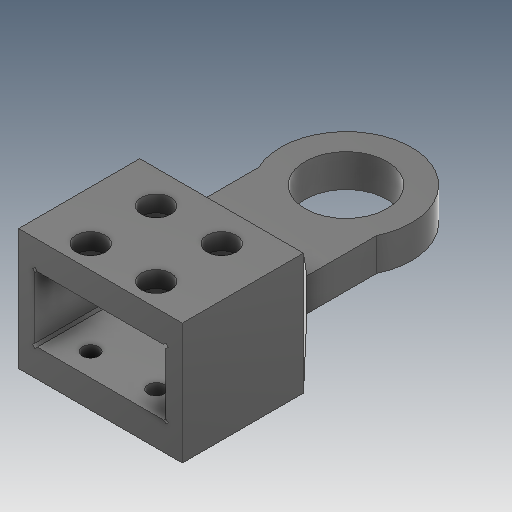
# Autodesk Inventor part: EndEffectorJoint
Saved by Autodesk Inventor 2020.3 (Build 243373000, 373)
## iProperties
Created: 2021-08-11
Part Number: EndEffectorJoint
Material: ABS Plastic
Document SubType Name: Modeling
Designer: justi
Density: 1.06 g/cm^3
Appearance: Smooth - Black
Mass: 59.7903 g
Surface Area: 233.875 cm^2
Volume: 56.4059 cm^3
Author: justi
Autodesk Inventor part; units mm, degrees
note: some values were not read from the file. Chosen so that the rebuilt part matches the saved one: direction of "Hole1".
ref_plane "YZ Plane" through (0, 0, 0) normal (1, 0, 0) x (0, 1, 0)
ref_plane "XZ Plane" through (0, 0, 0) normal (0, 1, 0) x (-1, 0, 0)
ref_plane "XY Plane" through (0, 0, 0) normal (0, 0, 1) x (1, 0, 0)
sketch "Sketch1" plane through (0, 0, 0) normal (0, 1, 0) x (-1, 0, 0)
  line L0 (25, 18.5) -> (-25, 18.5)
  line L1 (-25, 18.5) -> (-25, -18.5)
  line L2 (-25, -18.5) -> (25, -18.5)
  line L3 (25, -18.5) -> (25, 18.5)
  line L4 (25, 18.5) -> (-25, -18.5) construction
  line L5 (-25, 18.5) -> (25, -18.5) construction
  point P0 (0, 0)
  dimension "d0" = 50
  dimension "d1" = 37
  constraints: 12 end point, 2 midpoint, 2 parallel, 1 horizontal, 1 perpendicular
  measures "d0" distance of L2.end L1.end
  measures "d1" distance of L1.end L0.end
extrude "Extrusion1" add sketch "Sketch1" along normal mid plane 37
sketch "Sketch2" plane through (-25, 18.5, 18.5) normal (0, 0, 1) x (1, 0, 0)
  line L0 (5, -8.5) -> (45, -8.5)
  line L1 (45, -8.5) -> (45, -28.5)
  line L2 (45, -28.5) -> (5, -28.5)
  line L3 (5, -28.5) -> (5, -8.5)
  line L4 (5, -8.5) -> (45, -28.5) construction
  line L5 (45, -8.5) -> (5, -28.5) construction
  line L6 (5, -7.7929) -> (5.7071, -8.5)
  line L7 (5.7071, -8.5) -> (5, -9.2071)
  line L8 (5, -9.2071) -> (4.2929, -8.5)
  line L9 (4.2929, -8.5) -> (5, -7.7929)
  line L10 (4.5, -8) -> (5.5, -9) construction
  line L11 (5.5, -8) -> (4.5, -9) construction
  line L12 (45, -7.7929) -> (45.7071, -8.5)
  line L13 (45.7071, -8.5) -> (45, -9.2071)
  line L14 (45, -9.2071) -> (44.2929, -8.5)
  line L15 (44.2929, -8.5) -> (45, -7.7929)
  line L16 (45, -27.7929) -> (45.7071, -28.5)
  line L17 (45.7071, -28.5) -> (45, -29.2071)
  line L18 (45, -29.2071) -> (44.2929, -28.5)
  line L19 (44.2929, -28.5) -> (45, -27.7929)
  line L20 (5, -27.7929) -> (5.7071, -28.5)
  line L21 (5.7071, -28.5) -> (5, -29.2071)
  line L22 (5, -29.2071) -> (4.2929, -28.5)
  line L23 (4.2929, -28.5) -> (5, -27.7929)
  point P0 (25, -18.5)
  point P1 (5, -9.2071)
  point P2 (5, -27.7929)
  point P3 (5.7071, -28.5)
  point P4 (5.7071, -8.5)
  dimension "d4" = 40
  dimension "d5" = 20
  dimension "d6" = 1
  dimension "d7" = 1
  dimension "d8" = 1
  dimension "d9" = 1
  dimension "d10" = 1
  dimension "d11" = 1
  dimension "d12" = 1
  dimension "d13" = 1
  constraints: 48 end point, 10 parallel, 5 perpendicular, 4 midpoint, 1 horizontal
  measures "d4" distance of L1.end L2.end
  measures "d5" distance of L0.end L1.end
  measures "d6" distance of L7.end L8.end
  measures "d7" distance of L6.end L7.end
  measures "d8" distance of L14.start L14.end
  measures "d9" distance of L13.start L14.start
  measures "d10" distance of L18.start L18.end
  measures "d11" distance of L17.start L18.start
  measures "d12" distance of L22.start L22.end
  measures "d13" distance of L21.start L22.start
extrude "Extrusion2" cut sketch "Sketch2" against normal blind 37
sketch "Sketch3" plane through (0, 18.5, 0) normal (0, 1, 0) x (1, 0, 0)
  line L0 (25, -18.5) -> (-25, -18.5) construction
  line L1 (0, -18.5) -> (0, -1.5) construction
  line L2 (-10, 8.5) -> (10, 8.5) construction
  line L3 (10, 8.5) -> (10, -11.5) construction
  line L4 (10, -11.5) -> (-10, -11.5) construction
  line L5 (-10, -11.5) -> (-10, 8.5) construction
  line L6 (-10, 8.5) -> (10, -11.5) construction
  line L7 (10, 8.5) -> (-10, -11.5) construction
  point P0 (0, 0)
  dimension "d16" = 17
  dimension "d17" = 20
  dimension "d18" = 20
  constraints: 14 end point, 3 midpoint, 2 parallel, 1 horizontal, 1 perpendicular, 1 vertical
  measures "d16" distance of L1.start L1.end
  measures "d17" distance of L3.end L4.end
  measures "d18" distance of L2.end L3.end
hole "Hole1" at (-10, 18.5, 11.5) at (-10, 18.5, -8.5) at (10, 18.5, -8.5) at (10, 18.5, 11.5) direction (0, -1, 0) diameter 5 depth 8.5 counterbore diameter 9 counterbore depth 5
mirror "Mirror1" about plane through (0, 0, 0) normal (0, 1, 0) of "Hole1"
sketch "Sketch4" plane through (0, 0, 0) normal (0, 1, 0) x (-1, 0, 0)
  line L0 (19.2929, -18.5) -> (-19.2929, -18.5) projected
  line L1 (0, -18.5) -> (0, -56.5) construction
  line L2 (-25, -18.5) -> (25, -18.5) projected
  line L3 (25, 18.5) -> (25, -18.5) construction
  line L4 (0, -94.5) -> (0, -18.5) construction
  circle A0 centre (0, -56.5) radius 35
  line L5 (0, -21.5) -> (0, -26.5)
  line L6 (0, -26.5) -> (-18.0278, -26.5)
  line L7 (0, -26.5) -> (18.0278, -26.5)
  line L8 (-18.0278, -26.5) -> (-18.0278, -86.5)
  line L9 (18.0278, -26.5) -> (18.0278, -86.5)
  circle A1 centre (0, -56.5) radius 20
  point P0 (0, 0)
  point P1 (18.0278, -47.8397)
  point P2 (-18.0278, -47.8397)
  point P3 (-18.0278, -65.1603)
  point P4 (18.0278, -65.1603)
  dimension "d26" = 38
  dimension "d35" = 70
  dimension "d36" = 5
  dimension "d46" = 40
  constraints: 14 end point, 5 point on circle, 2 centre point, 2 coincident, 2 midpoint, 2 point on line, 2 vertical, 1 collinear, 1 horizontal, 1 perpendicular
  measures "d26" distance of L1.start L1.end
  measures "d35" diameter of A0
  measures "d36" distance of L5.start L5.end
  measures "d46" diameter of A1
extrude "Extrusion5" add sketch "Sketch4" along normal mid plane 10 contours L9 A1 L8 L6 L7 | A1 L9 | L9 A1 L8 | L8 A1
loft "Loft1" add separate body section 1 edges at (-25, 0, -18.5) (0, 18.5, -18.5) (25, 0, -18.5) (0, -18.5, -18.5) section 2 edges at (18.0278, 0, -26.5) (0, 5, -26.5) (-18.0278, 0, -26.5) (0, -5, -26.5)
sketch "Sketch6" plane through (0, 5, 0) normal (0, 1, 0) x (1, 0, 0)
  arc A0 (18.0278, 26.5) -> (-18.0278, 26.5) centre (0, 56.5) ccw projected
  circle A1 centre (0, 56.5) radius 12.5
  point P0 (0, 0)
  dimension "d43" = 25
  constraints: 2 coincident, 1 centre point
  measures "d43" diameter of A1
extrude "Extrusion6" cut sketch "Sketch6" against normal blind 10 bodies 1
body "Solid1"
body "Solid2"
